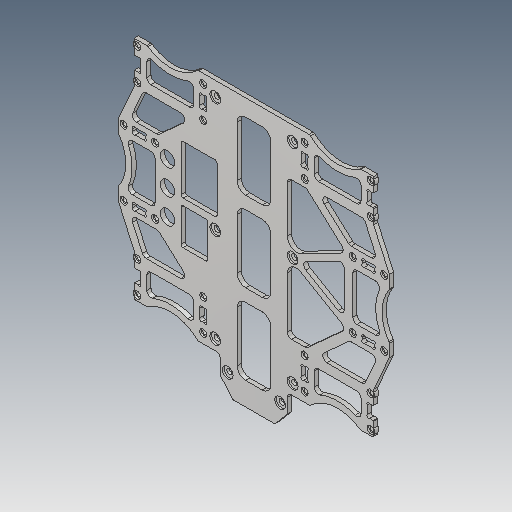
# Autodesk Inventor part: body_bottom
Saved by Autodesk Inventor 2019.4 (Build 234330000, 330)
## iProperties
Created: 2018-08-08
Part Number: body_bottom
Material: 一般
Document SubType Name: Modeling
Designer: student
Density: 1 g/cm^3
Appearance: 機械加工 - アルミニウム
Mass: 14.2227 g
Surface Area: 190.865 cm^2
Volume: 14.2227 cm^3
Author: student
Autodesk Inventor part; units mm, degrees
ref_plane "YZ Plane" through (0, 0, 0) normal (1, 0, 0) x (0, 1, 0)
ref_plane "XZ Plane" through (0, 0, 0) normal (0, 1, 0) x (-1, 0, 0)
ref_plane "XY Plane" through (0, 0, 0) normal (0, 0, 1) x (1, 0, 0)
sketch "スケッチ1" plane through (0, 0, 0) normal (0, 0, 1) x (1, 0, 0)
  arc A0 (80, 0) -> (40, 69.282) centre (0, 0) ccw construction
  line L0 (0, 0) -> (40, 69.282) construction
  line L1 (0, 0) -> (47.25, 0) construction
  arc A1 (56.2792, 52.132) -> (55.2208, 52.132) centre (55.75, 51.532) ccw construction
  arc A2 (56.2792, 37.132) -> (55.2208, 37.132) centre (55.75, 36.532) ccw construction
  arc A3 (24.7792, 52.132) -> (23.7208, 52.132) centre (24.25, 51.532) ccw construction
  arc A4 (24.7792, 37.132) -> (23.7208, 37.132) centre (24.25, 36.532) ccw construction
  circle A5 centre (24.25, 51.532) radius 1.05
  circle A6 centre (24.25, 36.532) radius 1.05
  circle A7 centre (55.75, 51.532) radius 1.05
  circle A8 centre (55.75, 36.532) radius 1.05
  line L2 (57.25, 54.032) -> (51.25, 54.032)
  line L3 (54.25, 54.032) -> (57.25, 54.032) construction
  line L4 (57.25, 52.132) -> (57.25, 53.782) construction
  line L5 (54.25, 47.032) -> (57.25, 47.032) construction
  line L6 (57.25, 41.032) -> (54.25, 41.032) construction
  line L7 (57.25, 34.032) -> (54.25, 34.032) construction
  line L8 (57.25, 54.032) -> (57.25, 52.8549)
  line L9 (57.25, 47.082) -> (55.2607, 47.082)
  line L10 (54.2, 47.082) -> (54.2, 46.0214) construction
  line L11 (54.2, 40.982) -> (55.2607, 40.982) construction
  line L12 (57.25, 40.982) -> (57.25, 37.8549)
  arc A9 (55.2607, 47.082) -> (54.2, 46.0214) centre (54.7303, 46.5517) ccw
  arc A10 (54.2, 42.0427) -> (55.2607, 40.982) centre (54.7303, 41.5124) ccw
  line L13 (55.2607, 47.082) -> (54.2, 47.082) construction
  line L14 (54.2, 46.0214) -> (54.2, 42.0427)
  line L15 (54.2, 42.0427) -> (54.2, 40.982) construction
  line L16 (55.2607, 40.982) -> (57.25, 40.982)
  line L17 (64.75, 14.25) -> (64.75, 17.25) construction
  line L18 (57.25, 34.032) -> (64.75, 17.25)
  line L19 (64.75, 17.25) -> (64.75, 11.25)
  arc A11 (27.0293, 55.7226) -> (50.6808, 53.8542) centre (40, 69.282) ccw
  arc A12 (64.5722, 10.6808) -> (64.5722, -10.6808) centre (80, 0) ccw
  line L20 (25.75, 54.032) -> (22.75, 54.032) construction
  arc A13 (51.25, 54.032) -> (50.6808, 53.8542) centre (51.25, 53.032) ccw
  arc A14 (27.0293, 55.7226) -> (26.3381, 56) centre (26.3381, 55) ccw
  line L21 (22.7, 40.982) -> (23.7607, 40.982) construction
  line L22 (25.8, 40.982) -> (25.8, 42.0427) construction
  line L23 (25.8, 47.082) -> (24.7393, 47.082) construction
  line L24 (22.7, 47.082) -> (22.7, 46.0214) construction
  line L25 (25.75, 46.782) -> (25.75, 41.282) construction
  line L26 (25.75, 47.032) -> (22.75, 47.032) construction
  line L27 (25.75, 41.032) -> (22.75, 41.032) construction
  line L28 (22.75, 41.282) -> (22.75, 46.782) construction
  arc A15 (22.7, 42.0427) -> (23.7607, 40.982) centre (23.2303, 41.5124) ccw
  arc A16 (23.7607, 47.082) -> (22.7, 46.0214) centre (23.2303, 46.5517) ccw
  arc A17 (25.8, 46.0214) -> (24.7393, 47.082) centre (25.2697, 46.5517) ccw
  arc A18 (24.7393, 40.982) -> (25.8, 42.0427) centre (25.2697, 41.5124) ccw
  line L29 (22.7, 46.0214) -> (22.7, 42.0427)
  line L30 (23.7607, 47.082) -> (22.7, 47.082) construction
  line L31 (24.7393, 47.082) -> (23.7607, 47.082)
  line L32 (25.8, 46.0214) -> (25.8, 47.082) construction
  line L33 (24.7393, 40.982) -> (25.8, 40.982) construction
  line L34 (25.8, 42.0427) -> (25.8, 46.0214)
  line L35 (23.7607, 40.982) -> (24.7393, 40.982)
  line L36 (22.7, 42.0427) -> (22.7, 40.982) construction
  line L37 (0, 56) -> (0, 0)
  arc A19 (64.5722, 10.6808) -> (64.75, 11.25) centre (63.75, 11.25) ccw
  line L38 (57.8, 17.3) -> (56.7393, 17.3) construction
  line L39 (51.7, 17.3) -> (51.7, 16.2393) construction
  line L40 (51.7, 14.2) -> (52.7607, 14.2) construction
  line L41 (57.8, 14.2) -> (57.8, 15.2607) construction
  line L42 (57.5, 14.25) -> (52, 14.25) construction
  line L43 (52, 17.25) -> (57.5, 17.25) construction
  line L44 (51.75, 17.25) -> (51.75, 14.25) construction
  line L45 (57.75, 14.25) -> (57.75, 17.25) construction
  arc A20 (52.7607, 17.3) -> (51.7, 16.2393) centre (52.2303, 16.7697) ccw
  arc A21 (51.7, 15.2607) -> (52.7607, 14.2) centre (52.2303, 14.7303) ccw
  arc A22 (56.7393, 14.2) -> (57.8, 15.2607) centre (57.2697, 14.7303) ccw
  arc A23 (57.8, 16.2393) -> (56.7393, 17.3) centre (57.2697, 16.7697) ccw
  line L46 (57.8, 16.2393) -> (57.8, 17.3) construction
  line L47 (56.7393, 17.3) -> (52.7607, 17.3)
  line L48 (57.8, 15.2607) -> (57.8, 16.2393)
  line L49 (56.7393, 14.2) -> (57.8, 14.2) construction
  line L50 (52.7607, 14.2) -> (56.7393, 14.2)
  line L51 (51.7, 15.2607) -> (51.7, 14.2) construction
  line L52 (51.7, 16.2393) -> (51.7, 15.2607)
  line L53 (52.7607, 17.3) -> (51.7, 17.3) construction
  arc A24 (62.85, 15.2208) -> (62.85, 16.2792) centre (62.25, 15.75) ccw construction
  circle A25 centre (62.25, 15.75) radius 1.05
  arc A26 (47.85, 15.2208) -> (47.85, 16.2792) centre (47.25, 15.75) ccw construction
  circle A27 centre (47.25, 15.75) radius 1.05
  line L54 (46.5207, 19.8) -> (56.1447, 19.8)
  line L55 (57.9706, 22.616) -> (53.2861, 33.0981)
  arc A28 (56.1447, 19.8) -> (57.9706, 22.616) centre (56.1447, 21.8) ccw
  arc A29 (31.5743, 49.2149) -> (48.4257, 49.2149) centre (40, 69.282) ccw
  line L56 (28.8, 47.3709) -> (28.8, 40.782)
  line L57 (30.8, 38.782) -> (49.2, 38.782)
  line L58 (51.2, 40.782) -> (51.2, 47.3709)
  arc A30 (31.5743, 49.2149) -> (28.8, 47.3709) centre (30.8, 47.3709) ccw
  arc A31 (51.2, 47.3709) -> (48.4257, 49.2149) centre (49.2, 47.3709) ccw
  arc A32 (49.2, 38.782) -> (51.2, 40.782) centre (49.2, 40.782) ccw
  arc A33 (28.8, 40.782) -> (30.8, 38.782) centre (30.8, 40.782) ccw
  line L59 (24.25, 36.532) -> (47.25, 15.75) construction
  line L60 (34.9199, 34.282) -> (51.4602, 34.282)
  line L61 (45.1798, 20.316) -> (33.5791, 30.7981)
  line L62 (54.3774, 36.532) -> (35.8774, 36.532) construction
  arc A34 (34.9199, 34.282) -> (33.5791, 30.7981) centre (34.9199, 32.282) ccw
  circle A35 centre (47.25, -15.75) radius 1.05 construction
  line L63 (47.25, -9.2) -> (47.25, 9.2)
  line L64 (49.25, 11.2) -> (58.0888, 11.2)
  arc A36 (59.9329, 8.4257) -> (59.9329, -8.4257) centre (80, 0) ccw
  arc A37 (49.25, 11.2) -> (47.25, 9.2) centre (49.25, 9.2) ccw
  arc A38 (59.9329, 8.4257) -> (58.0888, 11.2) centre (58.0888, 9.2) ccw
  line L65 (47.25, 0) -> (58.2358, 0) construction
  line L66 (58.2358, 0) -> (80, 0) construction
  line L67 (47.25, 0) -> (58.2358, 0) construction
  arc A39 (53.2861, 33.0981) -> (51.4602, 34.282) centre (51.4602, 32.282) ccw
  arc A40 (45.1798, 20.316) -> (46.5207, 19.8) centre (46.5207, 21.8) ccw
  line L68 (47.25, 15.75) -> (47.25, 0) construction
  line L69 (26.3381, 56) -> (0, 56)
  circle A41 centre (24.25, -51.532) radius 1.05
  circle A42 centre (24.25, -36.532) radius 1.05
  circle A43 centre (55.75, -36.532) radius 1.05
  line L70 (57.25, -54.032) -> (51.25, -54.032)
  line L71 (57.25, -47.082) -> (55.2607, -47.082)
  arc A44 (54.2, -46.0214) -> (55.2607, -47.082) centre (54.7303, -46.5517) ccw
  arc A45 (55.2607, -40.982) -> (54.2, -42.0427) centre (54.7303, -41.5124) ccw
  line L72 (54.2, -46.0214) -> (54.2, -42.0427)
  line L73 (55.2607, -40.982) -> (57.25, -40.982)
  arc A46 (50.6808, -53.8542) -> (27.0293, -55.7226) centre (40, -69.282) ccw
  arc A47 (50.6808, -53.8542) -> (51.25, -54.032) centre (51.25, -53.032) ccw
  arc A48 (26.3381, -56) -> (27.0293, -55.7226) centre (26.3381, -55) ccw
  line L74 (22.7, -40.982) -> (23.7607, -40.982) construction
  line L75 (25.8, -40.982) -> (25.8, -42.0427) construction
  line L76 (25.8, -47.082) -> (24.7393, -47.082) construction
  line L77 (22.7, -47.082) -> (22.7, -46.0214) construction
  arc A49 (23.7607, -40.982) -> (22.7, -42.0427) centre (23.2303, -41.5124) ccw
  arc A50 (22.7, -46.0214) -> (23.7607, -47.082) centre (23.2303, -46.5517) ccw
  arc A51 (24.7393, -47.082) -> (25.8, -46.0214) centre (25.2697, -46.5517) ccw
  arc A52 (25.8, -42.0427) -> (24.7393, -40.982) centre (25.2697, -41.5124) ccw
  line L78 (22.7, -46.0214) -> (22.7, -42.0427)
  line L79 (23.7607, -47.082) -> (22.7, -47.082) construction
  line L80 (24.7393, -47.082) -> (23.7607, -47.082)
  line L81 (25.8, -46.0214) -> (25.8, -47.082) construction
  line L82 (24.7393, -40.982) -> (25.8, -40.982) construction
  line L83 (25.8, -42.0427) -> (25.8, -46.0214)
  line L84 (23.7607, -40.982) -> (24.7393, -40.982)
  line L85 (22.7, -42.0427) -> (22.7, -40.982) construction
  arc A53 (64.75, -11.25) -> (64.5722, -10.6808) centre (63.75, -11.25) ccw
  line L86 (57.8, -17.3) -> (56.7393, -17.3) construction
  line L87 (51.7, -17.3) -> (51.7, -16.2393) construction
  line L88 (51.7, -14.2) -> (52.7607, -14.2) construction
  line L89 (57.8, -14.2) -> (57.8, -15.2607) construction
  arc A54 (51.7, -16.2393) -> (52.7607, -17.3) centre (52.2303, -16.7697) ccw
  arc A55 (52.7607, -14.2) -> (51.7, -15.2607) centre (52.2303, -14.7303) ccw
  arc A56 (57.8, -15.2607) -> (56.7393, -14.2) centre (57.2697, -14.7303) ccw
  arc A57 (56.7393, -17.3) -> (57.8, -16.2393) centre (57.2697, -16.7697) ccw
  line L90 (57.8, -16.2393) -> (57.8, -17.3) construction
  line L91 (56.7393, -17.3) -> (52.7607, -17.3)
  line L92 (57.8, -15.2607) -> (57.8, -16.2393)
  line L93 (56.7393, -14.2) -> (57.8, -14.2) construction
  line L94 (52.7607, -14.2) -> (56.7393, -14.2)
  line L95 (51.7, -15.2607) -> (51.7, -14.2) construction
  line L96 (51.7, -16.2393) -> (51.7, -15.2607)
  line L97 (52.7607, -17.3) -> (51.7, -17.3) construction
  circle A58 centre (62.25, -15.75) radius 1.05
  circle A59 centre (47.25, -15.75) radius 1.05
  line L98 (46.5207, -19.8) -> (56.1447, -19.8)
  line L99 (57.9706, -22.616) -> (53.2861, -33.0981)
  arc A60 (57.9706, -22.616) -> (56.1447, -19.8) centre (56.1447, -21.8) ccw
  arc A61 (48.4257, -49.2149) -> (31.5743, -49.2149) centre (40, -69.282) ccw
  line L100 (28.8, -47.3709) -> (28.8, -40.782)
  line L101 (30.8, -38.782) -> (49.2, -38.782)
  line L102 (51.2, -40.782) -> (51.2, -47.3709)
  arc A62 (28.8, -47.3709) -> (31.5743, -49.2149) centre (30.8, -47.3709) ccw
  arc A63 (48.4257, -49.2149) -> (51.2, -47.3709) centre (49.2, -47.3709) ccw
  arc A64 (51.2, -40.782) -> (49.2, -38.782) centre (49.2, -40.782) ccw
  arc A65 (30.8, -38.782) -> (28.8, -40.782) centre (30.8, -40.782) ccw
  line L103 (34.9199, -34.282) -> (51.4602, -34.282)
  line L104 (45.1798, -20.316) -> (33.5791, -30.7981)
  arc A66 (33.5791, -30.7981) -> (34.9199, -34.282) centre (34.9199, -32.282) ccw
  line L105 (49.25, -11.2) -> (58.0888, -11.2)
  arc A67 (47.25, -9.2) -> (49.25, -11.2) centre (49.25, -9.2) ccw
  arc A68 (58.0888, -11.2) -> (59.9329, -8.4257) centre (58.0888, -9.2) ccw
  arc A69 (51.4602, -34.282) -> (53.2861, -33.0981) centre (51.4602, -32.282) ccw
  arc A70 (46.5207, -19.8) -> (45.1798, -20.316) centre (46.5207, -21.8) ccw
  line L106 (26.3381, -56) -> (18, -56)
  circle A71 centre (18.5, -51) radius 1.3
  line L107 (0, -72) -> (10, -72)
  line L108 (10, -72) -> (16, -65)
  line L109 (16, -65) -> (16, -58)
  arc A72 (18, -56) -> (16, -58) centre (18, -58) ccw
  line L110 (0, -72) -> (0, 0)
  circle A73 centre (55.75, -51.532) radius 1.05
  circle A74 centre (12.5, -62) radius 1.3
  arc A75 (57.25, 50.2092) -> (57.25, 52.8549) centre (55.75, 51.532) ccw
  line L111 (57.25, 52.8549) -> (57.25, 50.2092) construction
  line L112 (57.25, 50.2092) -> (57.25, 47.082)
  arc A76 (57.25, 35.2092) -> (57.25, 37.8549) centre (55.75, 36.532) ccw
  line L113 (57.25, 37.8549) -> (57.25, 35.2092) construction
  line L114 (57.25, 35.2092) -> (57.25, 34.032)
  arc A77 (57.25, -52.8549) -> (57.25, -50.2092) centre (55.75, -51.532) ccw
  arc A78 (57.25, -37.8549) -> (57.25, -35.2092) centre (55.75, -36.532) ccw
  line L115 (57.25, -40.982) -> (57.25, -37.8549)
  line L116 (57.25, -35.2092) -> (57.25, -34.032)
  line L117 (57.25, -54.032) -> (57.25, -52.8549)
  line L118 (57.25, -50.2092) -> (57.25, -47.082)
  line L119 (57.25, -34.032) -> (64.75, -17.25)
  line L120 (64.75, -17.25) -> (64.75, -11.25)
  arc A79 (61.65, 16.2792) -> (61.65, 15.2208) centre (62.25, 15.75) ccw construction
  circle A80 centre (18.5, -51) radius 2 construction
  circle A81 centre (12.5, -62) radius 2 construction
  circle A82 centre (18.5, 49) radius 2 construction
  circle A83 centre (18.5, 49) radius 1.3
  point P0 (50.9332, 54.032)
  point P1 (64.75, 10.9332)
  point P2 (55.2496, 28.7046)
  point P3 (52.0165, 19.8)
  point P4 (28.8, 50.6208)
  point P5 (51.2, 50.6208)
  point P6 (61.3388, 11.2)
  point P7 (32.9702, 25.9572)
  point P8 (45.25, 13.125)
  point P9 (0, -56)
  point P10 (55.2496, -28.7046)
  point P11 (52.0165, -19.8)
  point P12 (32.9702, -25.9572)
  dimension "d3" = 60
  dimension "d7" = 2.1
  dimension "d8" = 0.05
  dimension "d9" = 0.05
  dimension "d10" = 3.05
  dimension "d11" = 0.75
  dimension "d13" = 1
  dimension "d14" = 1
  dimension "d15" = 6
  dimension "d16" = 0.05
  dimension "d17" = 0.05
  dimension "d18" = 0.05
  dimension "d19" = 0.05
  dimension "d20" = 0.75
  dimension "d21" = 1
  dimension "d22" = 6
  dimension "d23" = 0.05
  dimension "d24" = 0.05
  dimension "d25" = 0.05
  dimension "d26" = 0.05
  dimension "d27" = 0.75
  dimension "d28" = 2.1
  dimension "d29" = 6.95
  dimension "d31" = 4
  dimension "d32" = 2.5
  dimension "d34" = 3
  dimension "d35" = 3
  dimension "d36" = 3
  dimension "d38" = 2
  dimension "d40" = 4.5
  dimension "d41" = 2
  dimension "d42" = 4
  dimension "d48" = 2
  dimension "d49" = 3
  dimension "d50" = 3
  dimension "d54" = 2
  dimension "d55" = 2
  dimension "d67" = 56
  dimension "d78" = 80
  dimension "d80" = 2
  dimension "d81" = 72
  dimension "d82" = 16
  dimension "d83" = 6
  dimension "d84" = 7
  dimension "d113" = 2
  dimension "d119" = 2.6
  constraints: 211 end point, 132 point on circle, 99 symmetric about line, 74 centre point, 37 parallel, 34 perpendicular, 28 tangent, 19 equal radius, 18 horizontal, 18 point on line, 14 collinear, 10 coincident, 10 vertical, 7 concentric, 1 midpoint, 37 other
  measures "d3" angle of L1 L0
  measures "d7" diameter of A8
  measures "d8" distance between parallel lines of L9 L5
  measures "d9" distance between parallel lines of L11 L6
  measures "d10" distance between parallel lines of L10 L8
  measures "d11" radius of A9
  measures "d13" radius of A13
  measures "d14" radius of A14
  measures "d15" distance of L2.start L2.end
  measures "d16" distance between parallel lines of L21 L27
  measures "d18" distance between parallel lines of L23 L26
  measures "d19" distance between parallel lines of L24 L28
  measures "d20" radius of A15
  measures "d21" radius of A19
  measures "d22" distance of L17.end L19.end
  measures "d23" distance between parallel lines of L40 L42
  measures "d24" distance between parallel lines of L39 L44
  measures "d25" distance between parallel lines of L38 L43
  measures "d26" distance between parallel lines of L41 L45
  measures "d27" radius of A20
  measures "d28" diameter of A25
  measures "d29" distance of L12.start L18.start
  measures "d31" distance between parallel lines of L18 L55
  measures "d32" distance between parallel lines of L47 L54
  measures "d34" radial gap between concentric circles of A29 A11
  measures "d35" distance between parallel lines of L14 L58
  measures "d36" distance between parallel lines of L56 L34
  measures "d38" radius of A30
  measures "d40" distance between parallel lines of L60 L57
  measures "d41" radius of A34
  measures "d42" diameter of L61 L59
  measures "d48" radius of A37
  measures "d49" radial gap between concentric circles of A12 A36
  measures "d50" distance between parallel lines of L50 L64
  measures "d54" radius of A39
  measures "d55" radius of A28
  measures "d67" distance of L37.start L0.start
  measures "d78" radius of A0
  measures "d80" radius of A72
  measures "d81" distance of L107.start L0.start
  measures "d82" distance between parallel lines of L110 L109
  measures "d83" distance from line of L109 L107.end
  measures "d84" distance from line of L107 L108.end
  measures "d113" radius of A75
  measures "d119" diameter of A71
extrude "押し出し1" add sketch "スケッチ1" along normal blind 2
chamfer "面取り1" distance 0.5 angle 45 1 edges at (57.25, -54.032, 1)
chamfer "面取り2" distance 0.25 angle 45 4 edges at (57.25, -40.982, 1) (57.25, -47.082, 1) (57.25, 40.982, 1) (57.25, 47.082, 1)
mirror "ミラー2" about plane through (0, 0, 0) normal (1, 0, 0) of "押し出し1", "面取り1", "面取り2"
sketch "スケッチ3" plane through (0, 0, 2) normal (0, 0, 1) x (1, 0, 0)
  circle A0 centre (-41.3, -12) radius 3.45
  circle A1 centre (-41.3, 0) radius 3.45
  circle A2 centre (-41.3, 12) radius 3.45
  line L0 (-37.85, -22) -> (-37.85, 22) construction
  line L1 (-44.75, 12.25) -> (-44.75, -12.25) construction
  circle A3 centre (47.25, 15.75) radius 1.05 construction
  arc A4 (16, 8.7246) -> (22.5141, 4.7453) centre (20.4725, 8.7246) ccw
  line L2 (22.5141, 4.7453) -> (41.5805, 14.5272)
  line L3 (42.0084, 17.7906) -> (25.7115, 32.516)
  line L4 (24.3706, 33.032) -> (18, 33.032)
  line L5 (16, 31.032) -> (16, 8.7246)
  arc A5 (18, 33.032) -> (16, 31.032) centre (18, 31.032) ccw
  arc A6 (25.7115, 32.516) -> (24.3706, 33.032) centre (24.3706, 31.032) ccw
  arc A7 (41.5805, 14.5272) -> (42.0084, 17.7906) centre (40.6676, 16.3067) ccw
  line L6 (45.1798, 20.316) -> (33.5791, 30.7981) construction
  line L7 (34.9199, 34.282) -> (51.4602, 34.282) construction
  circle A8 centre (18.5, 1) radius 1.4
  line L8 (-4, 48) -> (4, 48)
  line L9 (8, 44) -> (8, 19.6667)
  line L10 (4, 15.6667) -> (-4, 15.6667)
  line L11 (-8, 19.6667) -> (-8, 44)
  line L12 (-4, 9.6667) -> (4, 9.6667)
  line L13 (8, 5.6667) -> (8, -18.6667)
  line L14 (4, -22.6667) -> (-4, -22.6667)
  line L15 (-8, -18.6667) -> (-8, 5.6667)
  line L16 (-4, -28.6667) -> (4, -28.6667)
  line L17 (8, -32.6667) -> (8, -57)
  line L18 (4, -61) -> (-4, -61)
  line L19 (-8, -57) -> (-8, -32.6667)
  arc A9 (-4, -28.6667) -> (-8, -32.6667) centre (-4, -32.6667) ccw
  arc A10 (8, -32.6667) -> (4, -28.6667) centre (4, -32.6667) ccw
  arc A11 (4, -61) -> (8, -57) centre (4, -57) ccw
  arc A12 (-8, -57) -> (-4, -61) centre (-4, -57) ccw
  arc A13 (-8, -18.6667) -> (-4, -22.6667) centre (-4, -18.6667) ccw
  arc A14 (4, -22.6667) -> (8, -18.6667) centre (4, -18.6667) ccw
  arc A15 (8, 5.6667) -> (4, 9.6667) centre (4, 5.6667) ccw
  arc A16 (-4, 9.6667) -> (-8, 5.6667) centre (-4, 5.6667) ccw
  arc A17 (-8, 19.6667) -> (-4, 15.6667) centre (-4, 19.6667) ccw
  arc A18 (4, 15.6667) -> (8, 19.6667) centre (4, 19.6667) ccw
  arc A19 (8, 44) -> (4, 48) centre (4, 44) ccw
  arc A20 (-4, 48) -> (-8, 44) centre (-4, 44) ccw
  line L20 (0, 0) -> (0, 60.956) construction
  line L21 (26.3381, 56) -> (-26.3381, 56) construction
  line L22 (7, -66) -> (-7, -66) construction
  circle A21 centre (-18.5, -5.95) radius 1.4
  line L23 (40.3371, 10.5175) -> (24.8744, 2.5845)
  line L24 (24.7806, -0.9231) -> (40.2432, -9.9318)
  line L25 (43.25, -8.2037) -> (43.25, 8.738)
  arc A22 (43.25, 8.738) -> (40.3371, 10.5175) centre (41.25, 8.738) ccw
  arc A23 (40.2432, -9.9318) -> (43.25, -8.2037) centre (41.25, -8.2037) ccw
  arc A24 (24.8744, 2.5845) -> (24.7806, -0.9231) centre (25.7874, 0.805) ccw
  line L26 (47.25, -9.2) -> (47.25, 9.2) construction
  arc A25 (22.1904, -2.8861) -> (16, -6.4438) centre (20.1176, -6.4438) ccw
  line L27 (22.1904, -2.8861) -> (41.9038, -14.3713)
  line L28 (42.2378, -17.5833) -> (25.7115, -32.516)
  line L29 (24.3706, -33.032) -> (18, -33.032)
  line L30 (16, -31.032) -> (16, -6.4438)
  arc A26 (16, -31.032) -> (18, -33.032) centre (18, -31.032) ccw
  arc A27 (24.3706, -33.032) -> (25.7115, -32.516) centre (24.3706, -31.032) ccw
  arc A28 (42.2378, -17.5833) -> (41.9038, -14.3713) centre (40.897, -16.0994) ccw
  arc A29 (19.5294, -2.3452) -> (19.5294, 4.3452) centre (18.5, 1) ccw construction
  line L31 (0, 0) -> (14.0478, 0) construction
  line L32 (47.25, 15.75) -> (18.5, 1) construction
  circle A30 centre (47.25, -15.75) radius 1.05 construction
  line L33 (18.5, 1) -> (47.25, -15.75) construction
  line L34 (33.5791, -30.7981) -> (45.1798, -20.316) construction
  line L35 (-41.3, 12) -> (-41.3, 0) construction
  line L36 (-41.3, 0) -> (-41.3, -12) construction
  line L37 (-41.3, 0) -> (0, 0) construction
  circle A31 centre (24.25, 36.532) radius 1.05 construction
  circle A32 centre (55.75, 36.532) radius 1.05 construction
  line L38 (24.25, 36.532) -> (55.75, 36.532) construction
  line L39 (-18.55, 0.55) -> (-33.85, 0.55) construction
  line L40 (-18.55, 22) -> (-18.55, 0.55) construction
  line L41 (-33.85, 22) -> (-18.55, 22) construction
  line L42 (-33.85, 0.55) -> (-33.85, 22) construction
  line L43 (-33.85, -20) -> (-33.85, -4.65) construction
  line L44 (-23, -20) -> (-33.85, -20) construction
  line L45 (-23, -4.65) -> (-23, -20) construction
  line L46 (-33.85, -4.65) -> (-23, -4.65) construction
  line L47 (-34.85, -20) -> (-34.85, -4.65)
  line L48 (-33.85, -3.65) -> (-23, -3.65)
  line L49 (-22, -4.65) -> (-22, -20)
  line L50 (-23, -21) -> (-33.85, -21)
  arc A33 (-33.85, -3.65) -> (-34.85, -4.65) centre (-33.85, -4.65) ccw
  arc A34 (-22, -4.65) -> (-23, -3.65) centre (-23, -4.65) ccw
  arc A35 (-23, -21) -> (-22, -20) centre (-23, -20) ccw
  arc A36 (-34.85, -20) -> (-33.85, -21) centre (-33.85, -20) ccw
  line L51 (-33.85, -0.45) -> (-18.55, -0.45)
  line L52 (-17.55, 0.55) -> (-17.55, 22)
  line L53 (-18.55, 23) -> (-33.85, 23)
  line L54 (-34.85, 22) -> (-34.85, 0.55)
  arc A37 (-18.55, -0.45) -> (-17.55, 0.55) centre (-18.55, 0.55) ccw
  arc A38 (-34.85, 0.55) -> (-33.85, -0.45) centre (-33.85, 0.55) ccw
  arc A39 (-33.85, 23) -> (-34.85, 22) centre (-33.85, 22) ccw
  arc A40 (-17.55, 22) -> (-18.55, 23) centre (-18.55, 22) ccw
  point P0 (-8, 9.6667)
  point P1 (8, -22.6667)
  point P2 (-8, -28.6667)
  point P3 (8, -61)
  point P4 (34.9199, -34.282)
  dimension "d89" = 2
  dimension "d90" = 4
  dimension "d95" = 2.8
  dimension "d97" = 8
  dimension "d98" = 5
  dimension "d99" = 6
  dimension "d100" = 6
  dimension "d101" = 16
  dimension "d115" = 2
  dimension "d117" = 4
  dimension "d120" = 2
  dimension "d121" = 3
  dimension "d122" = 3
  dimension "d123" = 32
  dimension "d124" = 4
  dimension "d125" = 4
  dimension "d126" = 12
  dimension "d127" = 3.5
  dimension "d128" = 1
  dimension "d129" = 1
  dimension "d130" = 1
  dimension "d131" = 1
  constraints: 78 end point, 66 tangent, 62 point on circle, 36 centre point, 26 equal radius, 12 point on line, 10 parallel, 6 horizontal, 4 collinear, 4 perpendicular, 4 vertical, 1 concentric, 10 other
  measures "d89" radius of A5
  measures "d90" distance between parallel lines of L6 L3
  measures "d95" diameter of A8
  measures "d97" distance between parallel lines of L21 L8
  measures "d98" distance between parallel lines of L18 L22
  measures "d99" distance between parallel lines of L12 L10
  measures "d100" distance between parallel lines of L16 L14
  measures "d101" distance between parallel lines of L9 L11
  measures "d115" radius of A24
  measures "d117" distance between parallel lines of L26 L25
  measures "d120" radius of A22
  measures "d121" distance between parallel lines of L23 L2
  measures "d122" distance between parallel lines of L27 L24
  measures "d123" diameter of L5 L20
  measures "d124" distance between parallel lines of L34 L28
  measures "d125" radius of A15
  measures "d126" distance of L35.end L36.end
  measures "d127" distance between parallel lines of L4 L38
  measures "d128" distance between parallel lines of L44 L50
  measures "d129" radius of A33
  measures "d130" distance between parallel lines of L39 L51
  measures "d131" radius of A37
extrude "押し出し3" cut sketch "スケッチ3" against normal blind 2
sketch "スケッチ4" plane through (0, 0, 2) normal (0, 0, 1) x (1, 0, 0)
  line L0 (0, 0) -> (0, -67.8124) construction
  circle A0 centre (55.75, 51.532) radius 1.05 projected
  circle A1 centre (55.75, 51.532) radius 1.7
  circle A2 centre (55.75, 36.532) radius 1.05 projected
  circle A3 centre (55.75, 36.532) radius 1.7
  circle A4 centre (24.25, 36.532) radius 1.05 projected
  circle A5 centre (24.25, 36.532) radius 1.7
  circle A6 centre (24.25, 51.532) radius 1.05 projected
  circle A7 centre (24.25, 51.532) radius 1.7
  circle A8 centre (62.25, 15.75) radius 1.05 projected
  circle A9 centre (62.25, 15.75) radius 1.7
  circle A10 centre (47.25, 15.75) radius 1.05 projected
  circle A11 centre (47.25, 15.75) radius 1.7
  circle A12 centre (47.25, -15.75) radius 1.05 projected
  circle A13 centre (47.25, -15.75) radius 1.7
  circle A14 centre (62.25, -15.75) radius 1.05 projected
  circle A15 centre (62.25, -15.75) radius 1.7
  line L1 (0, 0) -> (12.4062, 0) construction
  circle A16 centre (55.75, -51.532) radius 1.05
  circle A17 centre (55.75, -51.532) radius 1.7
  circle A18 centre (55.75, -36.532) radius 1.05
  circle A19 centre (55.75, -36.532) radius 1.7
  circle A20 centre (24.25, -36.532) radius 1.05
  circle A21 centre (24.25, -36.532) radius 1.7
  circle A22 centre (24.25, -51.532) radius 1.05
  circle A23 centre (24.25, -51.532) radius 1.7
  circle A24 centre (18.5, 1) radius 2.6
  circle A25 centre (18.5, -51) radius 1.3 projected
  circle A26 centre (18.5, -51) radius 2.6
  circle A27 centre (12.5, -62) radius 1.3 projected
  circle A28 centre (12.5, -62) radius 2.6
  circle A29 centre (-18.5, -51) radius 1.3
  circle A30 centre (-18.5, -51) radius 2.6
  circle A31 centre (-12.5, -62) radius 1.3
  circle A32 centre (-12.5, -62) radius 2.6
  circle A33 centre (-55.75, 51.532) radius 1.05
  circle A34 centre (-55.75, 51.532) radius 1.7
  circle A35 centre (-55.75, 36.532) radius 1.05
  circle A36 centre (-55.75, 36.532) radius 1.7
  circle A37 centre (-24.25, 36.532) radius 1.05
  circle A38 centre (-24.25, 36.532) radius 1.7
  circle A39 centre (-24.25, 51.532) radius 1.05
  circle A40 centre (-24.25, 51.532) radius 1.7
  circle A41 centre (-62.25, 15.75) radius 1.05
  circle A42 centre (-62.25, 15.75) radius 1.7
  circle A43 centre (-47.25, 15.75) radius 1.05
  circle A44 centre (-47.25, 15.75) radius 1.7
  circle A45 centre (-47.25, -15.75) radius 1.05
  circle A46 centre (-47.25, -15.75) radius 1.7
  circle A47 centre (-62.25, -15.75) radius 1.05
  circle A48 centre (-62.25, -15.75) radius 1.7
  circle A49 centre (-55.75, -36.532) radius 1.05
  circle A50 centre (-55.75, -36.532) radius 1.7
  circle A51 centre (-55.75, -51.532) radius 1.05
  circle A52 centre (-55.75, -51.532) radius 1.7
  circle A53 centre (-24.25, -36.532) radius 1.05
  circle A54 centre (-24.25, -36.532) radius 1.7
  circle A55 centre (-24.25, -51.532) radius 1.05
  circle A56 centre (-24.25, -51.532) radius 1.7
  circle A57 centre (-18.5, -5.95) radius 2.6
  circle A58 centre (18.5, 49) radius 1.3 projected
  circle A59 centre (-18.5, 49) radius 1.3 projected
  circle A60 centre (18.5, 49) radius 2.6
  circle A61 centre (-18.5, 49) radius 2.6
  circle A62 centre (18.5, 1) radius 1.4 projected
  circle A63 centre (-18.5, -5.95) radius 1.4 projected
  dimension "d109" = 3.4
  dimension "d110" = 5.2
  constraints: 50 centre point, 36 symmetric about line, 32 coincident, 12 equal radius, 4 end point, 2 concentric, 1 horizontal, 1 vertical, 36 other
  measures "d109" diameter of A3
  measures "d110" diameter of A24
extrude "押し出し4" cut sketch "スケッチ4" against normal blind 0.8 contours A0 | A1 | A2 | A3 | A4 | A5 | A6 | A7 | A8 | A9 | A10 | A11 | A12 | A13 | A14 | A15 | A16 | A17 | A18 | A19 | A20 | A21 | A22 | A23 | A24 | A25 | A26 | A27 | A28 | A29 | A30 | A31 | A32 | A33 | A34 | A35 | A36 | A37 | A38 | A39 | A40 | A41 | A42 | A43 | A44 | A45 | A46 | A47 | A48 | A49 | A50 | A51 | A52 | A53 | A54 | A55 | A56 | A57 | A60 | A61 | A62 | A63
